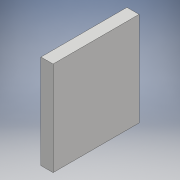
# Autodesk Inventor part: radiator 2018
Saved by Autodesk Inventor 2018.2 (Build 222227000, 227)
## iProperties
Created: 2018-05-19
Part Number: radiator 2018
Material: 一般
Document SubType Name: Modeling
Designer: ku_sk
Density: 1 g/cm^3
Appearance: 既定
Title: D:\ku_sk\ドキュメント\Inventor\Aero\KS-15\全体アッセンブリ解析用モデル\body\radiator\radiator 2018.stp
Author: ku_sk
Sending System: Autodesk Inventor 2018
Preprocessor: ST-DEVELOPER v17
Autodesk Inventor part; units mm, degrees
ref_plane "YZ Plane" through (0, 0, 0) normal (1, 0, 0) x (0, 1, 0)
ref_plane "XZ Plane" through (0, 0, 0) normal (0, 1, 0) x (-1, 0, 0)
ref_plane "XY Plane" through (0, 0, 0) normal (0, 0, 1) x (1, 0, 0)
sketch "スケッチ1" plane through (0, 0, 0) normal (1, 0, 0) x (0, 1, 0)
  line L0 (0, 0) -> (354.9654, 0)
  line L1 (354.9654, 0) -> (354.9654, 388.3801)
  line L2 (354.9654, 388.3801) -> (0, 388.3801)
  line L3 (0, 388.3801) -> (0, 0)
  constraints: 8 end point, 2 parallel, 1 horizontal, 1 perpendicular
extrude "押し出し1" add sketch "スケッチ1" along normal blind 50
